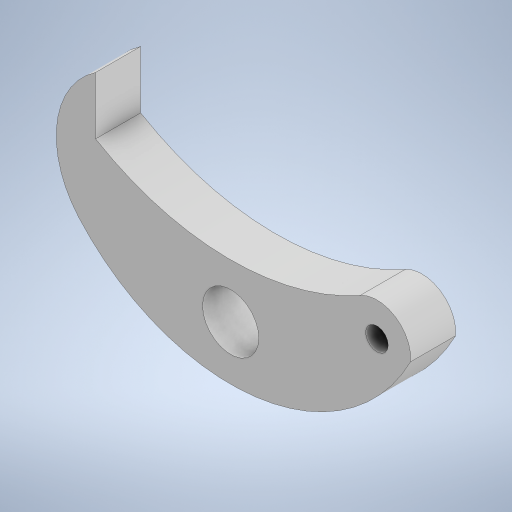
# Autodesk Inventor part: Hudson 1-66
Saved by Autodesk Inventor 2024.2 (Build 282272000, 272)
## iProperties
Created: 2024-10-10
Part Number: Hudson 1-66
Material: Generic
Document SubType Name: Modeling
Designer: Precisión-12
Density: 1 g/cm^3
Appearance: Default
Author: Precisión-12
Autodesk Inventor part; units mm, degrees
ref_plane "YZ Plane" through (0, 0, 0) normal (1, 0, 0) x (0, 1, 0)
ref_plane "XZ Plane" through (0, 0, 0) normal (0, 1, 0) x (-1, 0, 0)
ref_plane "XY Plane" through (0, 0, 0) normal (0, 0, 1) x (1, 0, 0)
sketch "Sketch1" plane through (0, 0, 0) normal (0, 0, 1) x (1, 0, 0)
  circle A0 centre (0, 0) radius 1.25
  line L0 (-13.143, 0) -> (13.143, 0) construction
  line L1 (0, 15.5803) -> (0, -15.5803) construction
  circle A1 centre (6.5, 2.6) radius 0.5
  arc A2 (7.9939, 2.4651) -> (5.7614, 3.9055) centre (6.5, 2.6) ccw
  arc A3 (-6, 4.0443) -> (5.7614, 3.9055) centre (0, 14.0887) ccw
  line L2 (-6, 6.6) -> (-6, 4.0443)
  arc A4 (-6.75, 0.6471) -> (7.9939, 2.4651) centre (0, 6.6) ccw
  arc A5 (-6, 6.6) -> (-6.021, 0) centre (-3.75, 3.2928) ccw
  dimension "d0" = 2.6
  dimension "d1" = 6.5
  dimension "d2" = 1.5
  dimension "d3" = 1
  dimension "d4" = 2.5
  dimension "d5" = 11.7
  dimension "d6" = 6
  dimension "d7" = 9
  dimension "d8" = 6.6
  dimension "d10" = 6.6
  dimension "d11" = 4
  constraints: 9 point on circle, 6 centre point, 6 end point, 3 coincident, 3 point on line, 2 midpoint, 2 vertical, 1 horizontal, 1 tangent
  measures "d0" distance from line of L0 A1.centre
  measures "d1" horizontal distance of point (0, 0) A1.centre
  measures "d2" radius of A2
  measures "d3" diameter of A1
  measures "d4" diameter of A0
  measures "d5" radius of A3
  measures "d6" distance between parallel lines of L1 L2
  measures "d7" radius of A4
  measures "d8" distance of point (0, 0) A4.centre
  measures "d10" distance from line of L0 L2.start
  measures "d11" radius of A5
extrude "Extrusion1" add sketch "Sketch1" along normal blind 2
body "Solid1"
